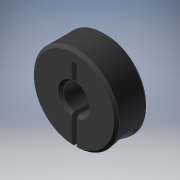
# Autodesk Inventor part: SSCSJ5-6b
Saved by Autodesk Inventor 2019 (Build 230136000, 136)
## iProperties
Created: 2022-10-17
Part Number: SSCSJ5-6b
Material: Generic
Catalog Web Link: www.cadenas.de
Description: SCSJ-b-Set Collars - Slit - Standard Compact Type
Vendor: MISUMI
Document SubType Name: Modeling
Designer: psAdmin
Manufacturer: MISUMI
Mass: 0.935244 g
Surface Area: 8.625 cm^2
Volume: 0.935244 cm^3
Density: 1 g/cm^3
Appearance: PSOLRGB-191-191-191
Category: PARTsolutions
Company: MISUMI
Title: SSCSJ5-6b
Author: Cadenas PARTsolutions
Comments: Set Collars - Slit - Standard Compact Type
PSOL_IDENT_0: {$CADENAS_DATA/23d-libs/misumi/metric/03_set_collars/scsj.prj},165 {VTYP=3D},{NB=SSCSJ5-6b},{LINA=SS
PSOL_IDENT_1: CSJ5-6b},{NN=SCSJ-b},{DATE=30.06.2021 12:51:58},{GEOMDATE=08.06.2021 01:39:00},{VERSION=},{LINEID=20
PSOL_IDENT_2: 0},{WBVAR=MAT,ST},{WBNUMERIC=}  {NB=SSCSJ5-6b},{LINA=SSCSJ5-6b},{KT=DUMMY},{PN=SSCSJ5-6},{TYPE=SSCSJ
PSOL_IDENT_3: },{MAT=2},{ST=},{STALG='','-'},{AC=Hexagon Socket Head Cap Screw 1 Pc. (SUS)},{D=5},{B=6},{D1=16},{M=
PSOL_IDENT_4: M2.6},{M1=2.6},{DD=2.9},{R=2.45},{W=1.00},{X=5.5},{Y=3},{Z=6.0},{C=0.5},{LS=6},{COLOR=0.75,0.75,0.75
PSOL_IDENT_5: ,0.00}
NB: SSCSJ5-6b
NN: SCSJ-b
NT: Set Collars - Slit - Standard Compact Type
NBSYN: $PN.b
LINA: SSCSJ5-6b
CATALOG: Misumi
PN: SSCSJ5-6
MAT: SUS304 Equivalent
ST: -
AC: Hexagon Socket Head Cap Screw 1 Pc. (SUS)
D: 5
B: 6
D1: 16
M: M2.6
DD: 2.9
R: 2.45
W: 1
X: 5.5
Y: 3
Z: 6
SUPPLIER: MISUMI
ARTICLENO: SSCSJ5-6b
BOMINFO: SSCSJ5-6b
CREATOR: CADENAS GmbH
Autodesk Inventor part; units mm, degrees
sketch "Sketch_1" plane through (0, 0, 0) normal (1, 0, 0) x (0, 1, 0)
  line L0 (0, -5) -> (0, 5)
  line L1 (7.5, 3) -> (3, 3)
  line L2 (3, 3) -> (2.5, 2.5)
  line L3 (2.5, 2.5) -> (2.5, -2.5)
  line L4 (2.5, -2.5) -> (3, -3)
  line L5 (3, -3) -> (7.5, -3)
  line L6 (7.5, -3) -> (8, -2.5)
  line L7 (8, -2.5) -> (8, 2.5)
  line L8 (8, 2.5) -> (7.5, 3)
  constraints: 18 end point
revolve "Revolution1" add sketch "Sketch_1" angle 360 about axis through (0, 0, -5) along (0, 0, 1)
sketch "Sketch_2" plane through (0, 0, 0) normal (0, 0, 1) x (1, 0, 0)
  line L0 (9.6, -5.5) -> (0.5, -5.5)
  line L1 (0.5, -5.5) -> (0.5, -4.05)
  line L2 (0.5, -4.05) -> (3, -4.05)
  line L3 (3, -4.05) -> (3, -3.05)
  line L4 (3, -3.05) -> (9.6, -3.05)
  line L5 (9.6, -3.05) -> (9.6, -5.5)
  line L6 (9.6, -5.5) -> (0.5, -5.5)
  constraints: 14 end point
revolve "Revolution2" cut sketch "Sketch_2" angle 360 about axis through (9.6, -5.5, 0) along (1, 0, 0)
sketch "Sketch_3" plane through (0, 0, 0) normal (0, 0, 1) x (1, 0, 0)
  line L0 (-0.5, -5.5) -> (-8, -5.5)
  line L1 (-8, -5.5) -> (-8, -4.4435)
  line L2 (-8, -4.4435) -> (-0.7435, -4.4435)
  line L3 (-0.7435, -4.4435) -> (-0.5, -4.2)
  line L4 (-0.5, -4.2) -> (-0.5, -5.5)
  line L5 (-0.5, -5.5) -> (-8, -5.5)
  constraints: 12 end point
revolve "Revolution3" cut sketch "Sketch_3" angle 360 about axis through (-0.5, -5.5, 0) along (1, 0, 0)
thread "Thread1" size "M2.6x0.45" class "6H" standard "ISO Metric profile" full length
sketch "Sketch_5" plane through (0, 0, 0) normal (0, 0, 1) x (1, 0, 0)
  line L0 (-0.5, 6) -> (-0.5, -9.6)
  line L1 (-0.5, -9.6) -> (0.5, -9.6)
  line L2 (0.5, -9.6) -> (0.5, 6)
  line L3 (0.5, 6) -> (-0.5, 6)
  constraints: 8 end point
extrude "Extrusion1" cut sketch "Sketch_5" along normal mid plane 6
ref_plane "to_screw_XY" through (3, -5.5, 0) normal (1, 0, 0) x (0, 0, -1)
ref_plane "to_screw_YZ" through (3, -5.5, 0) normal (0, 0, -1) x (0, 1, 0)
ref_plane "to_screw_ZX" through (3, -5.5, 0) normal (0, 1, 0) x (1, 0, 0)
body "Solid1"
